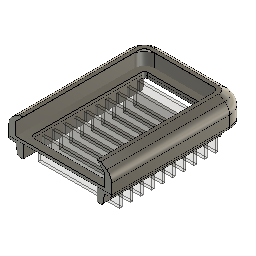
CRYSlight (Autodesk Fusion 360 design; units mm, degrees)
Autodesk Fusion 360 part; units mm, degrees
note: some values were not read from the file. Set by a fixed rule: which face or edge a step refers to.
sketch "clip" plane through (0, 0, 0) normal (0, 0, 1) x (1, 0, 0) in component "clip"
  line L0 (50, 72.5) -> (-50, 72.5)
  line L1 (-50, 72.5) -> (-50, -72.5)
  line L2 (-50, -72.5) -> (50, -72.5)
  line L3 (50, -72.5) -> (50, 72.5)
  line L4 (50, 72.5) -> (-50, -72.5) construction
  line L5 (-50, 72.5) -> (50, -72.5) construction
  line L6 (-42, -64.5) -> (42, -64.5)
  line L7 (42, -64.5) -> (42, 64.5)
  line L8 (42, 64.5) -> (-42, 64.5)
  line L9 (-42, 64.5) -> (-42, -64.5)
  line L10 (-58, 80.5) -> (-58, -80.5)
  line L11 (-58, -80.5) -> (58, -80.5)
  line L12 (58, -80.5) -> (58, 80.5)
  line L13 (58, 80.5) -> (-58, 80.5)
  line L14 (-42, -64.5) -> (-42, -80.5)
  line L15 (42, -64.5) -> (42, -80.5)
  line L16 (50, -72.5) -> (58, -72.5)
  line L17 (-50, -72.5) -> (-58, -72.5)
  line L18 (-42, -64.5) -> (-58, -64.5) construction
  line L19 (42, -64.5) -> (58, -64.5) construction
  line L20 (-50, -72.5) -> (-58, -64.5) construction
  line L21 (-58, -72.5) -> (-50, -64.5) construction
  line L22 (50, -72.5) -> (58, -64.5) construction
  line L23 (58, -72.5) -> (50, -64.5) construction
  circle A0 centre (-54, -68.5) radius 2
  circle A1 centre (54, -68.5) radius 2
  line L24 (42, 64.5) -> (50, 72.5) construction
  circle A2 centre (49.0711, 71.5711) radius 2
  line L25 (-42, 64.5) -> (-50, 72.5) construction
  circle A3 centre (-49.0711, 71.5711) radius 2
  line L26 (-42, 64.5) -> (-50, 64.5)
  line L27 (42, 64.5) -> (50, 64.5)
  line L28 (50, -51.5) -> (42, -51.5)
  line L29 (50, -48.5) -> (42, -48.5)
  line L30 (46, -51.5) -> (46, -48.5)
  dimension "d1" = 100
  dimension "d2" = 145
  dimension "d5" = -8
  dimension "d12" = 8
  dimension "d44" = 4
  dimension "d45" = 4
  dimension "d49" = 4
  dimension "d50" = 10
  dimension "d53" = 4
  dimension "d54" = 10
  dimension "d78" = 13
  dimension "d79" = 3
  dimension "d83" = 4
  constraint horizontal L0
  constraint perpendicular L0 L1
  constraint parallel L0 L2
  constraint parallel L1 L3
  constraint coincident L4 origin
  constraint coincident L5 origin
  constraint coincident L11 L14.end
  constraint perpendicular L11 L14
  constraint coincident L11 L15.end
  constraint perpendicular L11 L15
  constraint coincident L12 L16.end
  constraint perpendicular L12 L16
  constraint coincident L10 L17.end
  constraint perpendicular L10 L17
  constraint coincident L10 L18.end
  constraint perpendicular L10 L18
  constraint coincident L12 L19.end
  constraint perpendicular L12 L19
  constraint midpoint L18 L21.end
  constraint midpoint L19 L23.end
  constraint midpoint L21 A0.centre
  constraint midpoint L23 A1.centre
  constraint coincident L24 A2.centre
  constraint coincident L25 A3.centre
  constraint coincident L1 L26.end
  constraint perpendicular L1 L26
  constraint coincident L3 L27.end
  constraint perpendicular L3 L27
  constraint coincident L3 L28.start
  constraint coincident L7 L28.end
  constraint perpendicular L7 L28
  constraint coincident L3 L29.start
  constraint coincident L7 L29.end
  constraint perpendicular L7 L29
  constraint coincident L28 L30.start
  constraint coincident L29 L30.end
  constraint perpendicular L29 L30
  measures "d1" distance of L1.end L2.end
  measures "d2" distance of L0.end L1.end
  measures "d44" diameter of A0
  measures "d45" diameter of A1
  measures "d49" diameter of A2
  measures "d50" distance of L7.end A2.centre
  measures "d53" diameter of A3
  measures "d54" distance of L8.end A3.centre
  measures "d78" distance of L23.end L28.start
  measures "d79" distance of L28.start L29.start
  measures "d83" distance of L29.start L30.end
extrude "Extrude1" add sketch "clip" along normal blind 26 contours L0 L3 A2 | L0 L3 A2 | L0 L1 L3 L8 A2 A3 L26 L27 | L0 L1 L3 L10 L12 L13 L16 L17 A2 A3 | L0 L1 A3 | L0 L1 A3 | L3 L7 L27 L29 | L3 L28 L29 L30 | L6 L7 L8 L9 | L1 L2 L9 L14 L26 | L2 L3 L7 L15 L28 | L7 L28 L29 L30 | L2 L6 L14 L15 | A0 | A1 makes body 1 in component "clip"
extrude "Extrude3" cut sketch "clip" along normal blind 26 contours L6 L7 L8 L9 bodies 1 in component "clip"
extrude "Extrude4" cut sketch "clip" along normal blind 15 from surface at 3 contours L0 L3 A2 | L0 L1 L3 L8 A2 A3 L26 L27 | L0 L1 A3 | L3 L7 L27 L29 | L3 L28 L29 L30 | L1 L2 L9 L14 L26 | L2 L3 L7 L15 L28 | L7 L28 L29 L30 | L2 L6 L14 L15 picked at (48.4405, 70.9405) picked at (-48.4608, 70.9205) bodies 1 in component "clip"
extrude "Extrude7" cut sketch "clip" along normal blind 23 from surface at 3 contours L2 L6 L14 L15 bodies 1 in component "clip"
fillet "Fillet2" radius 12 2 edges at (50, 72.5, 10.5) (-50, 72.5, 10.5) on bodies 1 in component "clip"
fillet "Fillet2" radius 6 2 edges at (42, 64.5, 22) (-42, 64.5, 22) on bodies 1 in component "clip"
fillet "Fillet2" radius 20 2 edges at (58, 80.5, 13) (-58, 80.5, 13) on bodies 1 in component "clip"
fillet "Fillet2" radius 4 4 edges at (42, 64.5, 1.5) (-42, 64.5, 1.5) (-42, -64.5, 1.5) (42, -64.5, 1.5) on bodies 1 in component "clip"
extrude "Extrude8" cut sketch "clip" along normal blind 10 contours L0 L3 A2 | L0 L3 A2 | L0 L1 A3 | L0 L1 A3 | A0 | A1 bodies 1 in component "clip"
chamfer "Chamfer2" distance 7.95 angle 45 5 edges at (-42, -7, 18) (-40.2426, 62.7426, 18) (0, 64.5, 18) (40.2426, 62.7426, 18) (42, -7, 18) on bodies 1 in component "clip"
chamfer "Chamfer2" distance 12 distance2 8 5 edges at (58, -6, 26) (52.1421, 74.6421, 26) (0, 80.5, 26) (-52.1421, 74.6421, 26) (-58, -6, 26) measured on face at (-52.6667, 15.5, 26) measured on face at (38.9516, 80.4773, 8.6667) measured on face at (-52.6667, 15.5, 26) measured on face at (-38.9516, 80.4773, 8.6667) measured on face at (-52.6667, 15.5, 26) on bodies 1 in component "clip"
fillet "Fillet3" radius 12 5 edges at (58, -6, 18) (52.1421, 74.6421, 18) (0, 80.5, 18) (-52.1421, 74.6421, 18) (-58, -6, 18) on bodies 1 in component "clip"
extrude "Extrude4'" add sketch "clip" against normal blind 3 separate body contours L0 L1 L3 L8 A2 A3 L26 L27 | L0 L1 L3 L10 L12 L13 L16 L17 A2 A3 | L3 L7 L27 L29 | L3 L28 L29 L30 | L1 L2 L9 L14 L26 | L2 L3 L7 L15 L28 | L7 L28 L29 L30 makes body 2 in component "bracket"
extrude "Extrude5" add sketch "clip" against normal blind 15 contours L3 L7 L27 L29 | L3 L28 L29 L30 | L1 L2 L9 L14 L26 | L2 L3 L7 L15 L28 | L7 L28 L29 L30 bodies 2 in component "bracket"
fillet "Fillet2'" radius 20 2 edges at (-58, 80.5, -1.5) (58, 80.5, -1.5) on bodies 2 in component "bracket"
fillet "Fillet2'" radius 4 2 edges at (42, 64.5, -1.5) (-42, 64.5, -1.5) on bodies 2 in component "bracket"
chamfer "Chamfer1" distance 2 distance2 12 4 edges at (50, -4, -15) (-50, -4, -15) (46, 64.5, -15) (-46, 64.5, -15) measured on face at (44.6667, 18.8333, -15) measured on face at (-47.3333, 18.8333, -15) measured on face at (44.6667, 18.8333, -15) measured on face at (-47.3333, 18.8333, -15) on bodies 2 in component "bracket"
chamfer "Chamfer1" distance 1 angle 45 5 edges at (52.1421, 74.6421, -3) (58, -6, -3) (-58, -6, -3) (-52.1421, 74.6421, -3) (0, 80.5, -3) on bodies 2 in component "bracket"
fillet "Fillet3'" radius 2 6 edges at (-48, -5, -15) (48, -5, -15) (-49, 63.5, -9) (-45, 62.5, -15) (45, 62.5, -15) (49, 63.5, -9) on bodies 2 in component "bracket"
extrude "Extrude7'" cut sketch "clip" against normal blind 12 from surface at -3 contours L7 L28 L29 L30 bodies 2 in component "bracket"
mirror "Mirror1" about plane through (0, 0, 0) normal (1, 0, 0) of "Extrude7'" in component "bracket"
pattern_linear "R-Pattern1" count 10 spacing 12 along (0, 1, 0) of "Extrude7'", "Mirror1" in component "bracket"
extrude "Extrude1'" add 1 faces at (-46, -50.5, -7) along direction (1, 0, 0) blind 92 separate body on bodies 2 makes body 3 in component "shade"
extrude "Extrude2" add 1 faces at (-15.3333, -50.5, -15) along direction (0, 0, -1) blind 15 on bodies 3 bodies 3 in component "shade"
pattern_linear "R-Pattern1'" count 10 spacing 12 along (0, 1, 0) of bodies 3 makes body 4 at (-15.3333, -39.5, -12) makes body 5 at (-15.3333, -27.5, -12) makes body 6 at (-15.3333, -15.5, -12) makes body 7 at (-15.3333, -3.5, -12) makes body 8 at (-15.3333, 8.5, -12) makes body 9 at (-15.3333, 20.5, -12) makes body 10 at (-15.3333, 32.5, -12) makes body 11 at (-15.3333, 44.5, -12) makes body 12 at (-15.3333, 56.5, -12) in component "shade"
component "clip" placed x (1, 0, 0) y (0, 1, 0) z (0, 0, 1) at (0, 0, 0)
component "bracket" placed x (1, 0, 0) y (0, 1, 0) z (0, 0, 1) at (0, 0, 0)
component "shade" placed x (1, 0, 0) y (0, 1, 0) z (0, 0, 1) at (0, 0, 0)
named bodies: "clipBody", "bracketBody"
